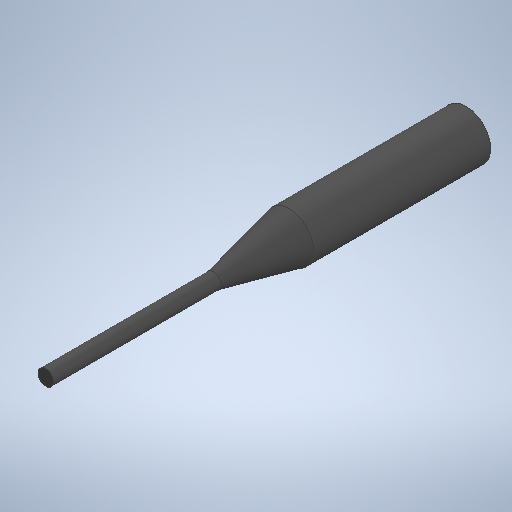
# Autodesk Inventor part: Microphone
Saved by Autodesk Inventor 2025 (Build 290162000, 162)
## iProperties
Created: 2024-09-06
Part Number: Microphone
Material: Generic
Document SubType Name: Modeling
Designer: Cupri
Density: 1 g/cm^3
Appearance: Default
Author: Cupri
Autodesk Inventor part; units mm, degrees
ref_plane "YZ Plane" through (0, 0, 0) normal (1, 0, 0) x (0, 1, 0)
ref_plane "XZ Plane" through (0, 0, 0) normal (0, 1, 0) x (-1, 0, 0)
ref_plane "XY Plane" through (0, 0, 0) normal (0, 0, 1) x (1, 0, 0)
sketch "Sketch1" plane through (0, 0, 0) normal (0, 1, 0) x (-1, 0, 0)
  line L0 (4, 109) -> (-4, 109)
  line L1 (-12.7, -17.2651) -> (-12.7, -109)
  line L2 (-12.7, -109) -> (12.7, -109)
  line L3 (12.7, -109) -> (12.7, -17.2651)
  line L4 (12.7, 109) -> (-12.7, -109) construction
  line L5 (-12.7, 109) -> (12.7, -109) construction
  line L6 (4, 22.0198) -> (12.7, -17.2651)
  line L7 (12.7, 109) -> (-12.7, -109) construction
  line L8 (-4, 22.0198) -> (-12.7, -17.2651)
  line L9 (4, 22.0198) -> (4, 109)
  line L10 (-4, 22.0198) -> (-4, 109)
  line L11 (0, 109) -> (0, -109)
  point P0 (0, 0)
  dimension "d0" = 25.4
  dimension "d1" = 218
  dimension "d9" = 8
  constraints: 24 end point, 4 midpoint, 3 perpendicular, 2 parallel, 1 horizontal
  measures "d0" distance of L1.end L2.end
  measures "d1" distance of L5.start L1.end
  measures "d9" distance between parallel lines of L10 L9
revolve "Revolution1" add sketch "Sketch1" angle 360 about axis through (0, 0, 109) along (0, 0, -1) contours L9 L6 L3 L2 L11 L0
body "Solid1"
